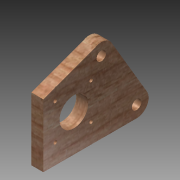
# Autodesk Inventor part: Y_MotorMount
Saved by Autodesk Inventor 2014 (Build 180170000, 170)
## iProperties
Created: 2013-12-16
Part Number: Y_MotorMount
Material: Birch
Document SubType Name: Modeling
Designer: Bram
Density: 0.512 g/cm^3
Appearance: Birch - Natural Medium Gloss
Author: Bram
Autodesk Inventor part; units mm, degrees
ref_plane "YZ Plane" through (0, 0, 0) normal (1, 0, 0) x (0, 1, 0)
ref_plane "XZ Plane" through (0, 0, 0) normal (0, 1, 0) x (-1, 0, 0)
ref_plane "XY Plane" through (0, 0, 0) normal (0, 0, 1) x (1, 0, 0)
sketch "Sketch1" plane through (0, 0, 0) normal (1, 0, 0) x (0, 1, 0)
  circle A0 centre (52.468, 74.8832) radius 4
  circle A1 centre (81.968, 24.8832) radius 4
  circle A2 centre (29.468, 45.8832) radius 12
  circle A3 centre (13.968, 61.3832) radius 1.5
  circle A4 centre (43.968, 61.3832) radius 1.5
  circle A5 centre (43.968, 31.3832) radius 1.5
  circle A6 centre (13.968, 31.3832) radius 1.5
  arc A7 (61.2976, 79.5777) -> (47.3885, 83.497) centre (52.468, 74.8832) ccw
  arc A8 (81.968, 14.8832) -> (90.2193, 30.5327) centre (81.968, 24.8832) ccw
  line L0 (60.8493, 80.3379) -> (90.9051, 29.3697)
  line L1 (47.3885, 83.497) -> (7.3003, 68.8293)
  line L2 (3.968, 61.3832) -> (3.968, 67.6101)
  line L3 (7.3003, 68.8293) -> (3.968, 67.6101)
  line L4 (3.968, 61.3832) -> (3.968, 14.8832)
  line L5 (81.968, 14.8832) -> (3.968, 14.8832)
  point P0 (0, 0)
  constraints: 12 end point, 9 centre point, 6 point on circle, 2 coincident, 2 collinear, 2 point on line, 1 tangent
extrude "Extrusion1" add sketch "Sketch1" along normal blind 10 contours L0 A8 L5 L4 L2 L3 L1 A7
body "Solid1"
